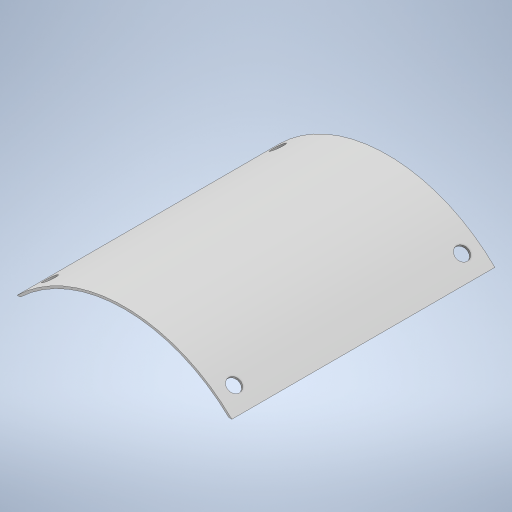
# Autodesk Inventor part: Electronics Door
Saved by Autodesk Inventor 2024 (Build 280153000, 153)
## iProperties
Created: 2024-04-23
Part Number: Electronics Door
Material: Generic
Document SubType Name: Modeling
Designer: auror
Density: 1 g/cm^3
Appearance: Default
Author: auror
Autodesk Inventor part; units mm, degrees
ref_plane "YZ Plane" through (0, 0, 0) normal (1, 0, 0) x (0, 1, 0)
ref_plane "XZ Plane" through (0, 0, 0) normal (0, 1, 0) x (-1, 0, 0)
ref_plane "XY Plane" through (0, 0, 0) normal (0, 0, 1) x (1, 0, 0)
sketch "Sketch8" plane through (0, 0, 0) normal (0, 0, 1) x (1, 0, 0)
  arc A0 (23.7678, 25.0068) -> (-23.7678, 25.0068) centre (0, 0) ccw
  arc A1 (24.495, 24.9999) -> (-24.495, 24.9999) centre (0, 0) ccw
  line L0 (-23.7678, 25.0068) -> (-24.495, 24.9999)
  line L1 (-24.6461, 24.172) -> (-22.9143, 25.818) construction
  line L2 (22.991, 25.7452) -> (24.5566, 24.2571) construction
  line L3 (23.7678, 25.0068) -> (24.495, 24.9999)
  line L4 (-24.495, 24.9999) -> (24.495, 24.9999) construction
  dimension "d88" = 34.5
  dimension "d89" = 35
  dimension "d90" = 0
  dimension "d91" = 137
  dimension "d92" = 0
  dimension "d93" = 137
  dimension "d98" = 48.99
  constraints: 10 end point, 4 point on circle, 2 centre point, 2 coincident, 2 tangent, 1 horizontal
  measures "d88" radius of A0
  measures "d89" radius of A1
  measures "d90" distance from line of L0.start L1
  measures "d91" angle of L0 L1
  measures "d92" distance from line of L3.start L2
  measures "d93" angle of L3 L2
  measures "d98" distance of L0.end L3.end
extrude "Extrusion5" add sketch "Sketch8" along normal blind 60
sketch "Sketch19" plane through (0, 0, 60) normal (0, 0, 1) x (1, 0, 0)
  line L0 (-24.495, 24.9999) -> (-23.7678, 25.0068) construction
  line L1 (-22.2755, 25.021) -> (-7.4699, 32.6566) construction
  arc A0 (22.2755, 25.021) -> (-22.2755, 25.021) centre (0, 0) ccw construction
  dimension "d162" = 32.448
  constraints: 2 end point, 1 point on circle
  measures "d162" distance from line of point (0, 0) L1
sketch "Sketch22" plane through (0, 0, 60) normal (0, 0, 1) x (1, 0, 0)
  line L0 (0, 0) -> (24.1157, 25.3728) construction
  line L1 (0, 0) -> (31.1859, 21.3976) construction
  arc A0 (23.7678, 25.0068) -> (-23.7678, 25.0068) centre (0, 0) ccw construction
  arc A1 (30.2355, 16.6152) -> (23.7678, 25.0068) centre (0, 0) ccw construction
  line L2 (28.4476, 19.5187) -> (9.8576, 33.0617) construction
  point P0 (19.8728, 25.7656)
  dimension "d175" = 12
  dimension "d176" = 23
  dimension "d177" = 0
  dimension "d178" = 10.609
  constraints: 6 end point, 4 point on circle, 2 point on line, 1 centre point, 1 coincident
  measures "d175" angle of L0 L1
  measures "d176" distance of L2.start L2.end
  measures "d177" distance from line of A0.start L0
  measures "d178" distance of L2.start point (19.873, 25.766)
sketch "Sketch23" plane through (0, 0, 0) normal (0, 0, -1) x (-1, 0, 0)
  arc A0 (23.7678, 25.0068) -> (-23.7678, 25.0068) centre (0, 0) ccw projected
  line L0 (0, 0) -> (-23.7678, 25.0068) construction
  line L1 (0, 0) -> (-30.9004, 21.2017) construction
  arc A1 (-23.7678, 25.0068) -> (-30.0627, 16.9258) centre (0, 0) ccw construction
  line L2 (-28.4476, 19.5187) -> (-9.8576, 33.0617) construction
  dimension "d179" = 12
  dimension "d180" = 23
  constraints: 6 end point, 4 point on circle, 1 centre point, 1 coincident, 1 point on line
  measures "d179" angle of L0 L1
  measures "d180" distance of L2.start L2.end
ref_plane "Work Plane12" through (28.4476, 19.5187, 60) normal (-0.5888245, -0.8082609, 0) x (-0.8082609, 0.5888245, 0)
sketch "Sketch24" plane through (28.4476, 19.5187, 60) normal (-0.5888245, -0.8082609, 0) x (-0.8082609, 0.5888245, 0)
  line L0 (7.014, 60) -> (7.014, 0) projected
  line L1 (45.4352, 0) -> (7.014, 0) projected
  line L2 (45.4352, 60) -> (7.014, 60) projected
  point P0 (11.5, 60)
  point P1 (11.014, 56)
  point P2 (11.014, 4)
  dimension "d181" = 4
  dimension "d182" = 4
  dimension "d183" = 4
  dimension "d184" = 4
  measures "d181" distance from line of L0 point (11.014, 4)
  measures "d182" distance from line of point (11.014, 4) L1
  measures "d183" distance from line of L2 point (11.014, 56)
  measures "d184" distance from line of L0 point (11.014, 56)
hole "Hole11" at (19.5454, 26.0041, 4) at (19.5454, 26.0041, 56) direction (0.5888245, 0.8082609, 0) diameter 3.1 end through all
ref_plane "Work Plane13" through (0, 25.2328, 0) normal (1, 0, 0) x (0, 0, 1)
mirror "Mirror2" about plane through (0, 25.2328, 0) normal (1, 0, 0) of "Hole11"
body "Solid2"
